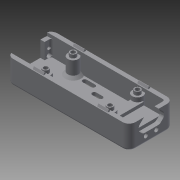
# Autodesk Inventor part: dualBaccable-ucan_fysect
Saved by Autodesk Inventor 2014 SP2 (Build 180246200, 246)
## iProperties
Created: 2025-01-14
Part Number: dualBaccable-ucan_fysect
Material: Generic
Document SubType Name: Sheet Metal
Designer: GauchoHP
Density: 1 g/cm^3
Sheet Metal Rule: Default_mm
Appearance: Default
Author: GauchoHP
Autodesk Inventor part; units mm, degrees
ref_plane "YZ Plane" through (0, 0, 0) normal (1, 0, 0) x (0, 1, 0)
ref_plane "XZ Plane" through (0, 0, 0) normal (0, 1, 0) x (-1, 0, 0)
ref_plane "XY Plane" through (0, 0, 0) normal (0, 0, 1) x (1, 0, 0)
sketch "Sketch1" plane through (0, 0, 0) normal (0, 0, 1) x (1, 0, 0)
  line L0 (-27.1053, 8.3421) -> (24.8947, 8.3421)
  line L1 (27.8947, 5.3421) -> (27.8947, -9.6579)
  line L2 (24.8947, -12.6579) -> (-27.1053, -12.6579)
  line L3 (-30.1053, -9.6579) -> (-30.1053, 5.3421)
  arc A0 (-27.1053, 8.3421) -> (-30.1053, 5.3421) centre (-27.1053, 5.3421) ccw
  arc A1 (27.8947, 5.3421) -> (24.8947, 8.3421) centre (24.8947, 5.3421) ccw
  arc A2 (24.8947, -12.6579) -> (27.8947, -9.6579) centre (24.8947, -9.6579) ccw
  arc A3 (-30.1053, -9.6579) -> (-27.1053, -12.6579) centre (-27.1053, -9.6579) ccw
  point P0 (0, 0)
  point P1 (-30.1053, 8.3421)
  point P2 (27.8947, 8.3421)
  point P3 (-30.1053, -12.6579)
  dimension "d0" = 21
  dimension "d1" = 58
  dimension "d2" = 3
  constraints: 8 end point, 8 point on circle, 8 tangent, 6 point on line, 4 centre point, 3 equal radius, 2 parallel, 1 horizontal, 1 perpendicular
  measures "d0" distance of point (-30.105, -12.658) point (-30.105, 8.342)
  measures "d1" distance of point (-30.105, 8.342) point (27.895, 8.342)
  measures "d2" radius of A0
extrude "Extrusion1" add sketch "Sketch1" along normal blind 2
sketch "Sketch2" plane through (0, 0, 2) normal (0, 0, 1) x (1, 0, 0)
  line L0 (24.8947, 8.3421) -> (-27.1053, 8.3421) projected
  arc A0 (-27.1053, 8.3421) -> (-30.1053, 5.3421) centre (-27.1053, 5.3421) ccw projected
  line L1 (-30.1053, 5.3421) -> (-30.1053, -9.6579) projected
  arc A1 (-30.1053, -9.6579) -> (-27.1053, -12.6579) centre (-27.1053, -9.6579) ccw projected
  line L2 (-27.1053, -12.6579) -> (24.8947, -12.6579) projected
  arc A2 (24.8947, -12.6579) -> (27.8947, -9.6579) centre (24.8947, -9.6579) ccw projected
  line L3 (27.8947, -9.6579) -> (27.8947, 5.3421) projected
  arc A3 (27.8947, 5.3421) -> (24.8947, 8.3421) centre (24.8947, 5.3421) ccw projected
  line L4 (-27.1053, 6.3421) -> (24.8947, 6.3421)
  arc A4 (25.8947, 5.3421) -> (24.8947, 6.3421) centre (24.8947, 5.3421) ccw
  line L5 (25.8947, 5.3421) -> (25.8947, -9.6579)
  arc A5 (24.8947, -10.6579) -> (25.8947, -9.6579) centre (24.8947, -9.6579) ccw
  line L6 (24.8947, -10.6579) -> (-27.1053, -10.6579)
  arc A6 (-28.1053, -9.6579) -> (-27.1053, -10.6579) centre (-27.1053, -9.6579) ccw
  line L7 (-28.1053, -9.6579) -> (-28.1053, 5.3421)
  arc A7 (-27.1053, 6.3421) -> (-28.1053, 5.3421) centre (-27.1053, 5.3421) ccw
  point P0 (0, 0)
  dimension "d5" = 2
  constraints: 8 end point, 8 point on circle, 4 centre point, 7 other
  measures "d5" distance between parallel lines of L4 L0
extrude "Extrusion2" add sketch "Sketch2" along normal blind 9.1
sketch "Sketch4" plane through (-28.1053, -9.6579, 2) normal (1, 0, 0) x (0, 0, -1)
  line L0 (0, 15) -> (0, 0) projected
  line L1 (0, 15) -> (-9.1, 15) projected
  line L2 (0, 0) -> (-9.1, 0) projected
  line L3 (0, 13) -> (-9.5, 13)
  line L4 (-9.5, 13) -> (-9.5, 0)
  line L5 (-9.5, 0) -> (0, 0)
  line L6 (0, 0) -> (0, 13)
  line L7 (-9.5, -1) -> (-7.5, -1)
  line L8 (-7.5, -1) -> (-7.5, 16)
  line L9 (-7.5, 16) -> (-9.5, 16)
  line L10 (-9.5, 16) -> (-9.5, -1)
  point P0 (2, 9.6579)
  dimension "d22" = 9.5
  dimension "d23" = 13
  dimension "d26" = 0
  dimension "d27" = 2
  dimension "d28" = 1
  dimension "d29" = 17
  dimension "d30" = 1
  dimension "d31" = 1
  dimension "d32" = 3
  dimension "d53" = 0
  constraints: 16 end point, 4 parallel, 2 horizontal, 2 perpendicular, 1 point on line
  measures "d22" distance of L5.end L4.end
  measures "d23" distance of L4.end L3.end
  measures "d26" distance between parallel lines of L5 L2
  measures "d27" distance of L8.end L9.end
  measures "d28" distance between parallel lines of L5 L7
  measures "d29" distance of L9.end L7.start
  measures "d30" distance between parallel lines of L9 L1
  measures "d31" distance between parallel lines of L2 L7
  measures "d32" distance between parallel lines of L9 L3
  measures "d53" distance between parallel lines of L4 L10
extrude "Extrusion4" cut sketch "Sketch4" along normal mid plane 10 contours L0 L2 L8 L3 | L8 L3 L10 L9 | L8 L2 L5 L4 L3 | L8 L7 L10 L5 L2
sketch "Sketch5" plane through (0, 0, 2) normal (0, 0, 1) x (1, 0, 0)
  line L0 (-27.1053, -10.6579) -> (24.8947, -10.6579) projected
  line L1 (25.8947, -9.6579) -> (25.8947, 5.3421) projected
  line L2 (24.8947, 6.3421) -> (-27.1053, 6.3421) projected
  line L3 (13.8947, 4.3421) -> (25.8947, 4.3421)
  line L4 (25.8947, 4.3421) -> (25.8947, -8.6579)
  line L5 (25.8947, -8.6579) -> (13.8947, -8.6579)
  line L6 (13.8947, -8.6579) -> (13.8947, 4.3421)
  line L7 (13.8947, -8.6579) -> (16.8947, -8.6579)
  line L8 (16.8947, -8.6579) -> (16.8947, -8.6579)
  line L9 (14.8947, -6.6579) -> (13.8947, -6.6579)
  line L10 (13.8947, -6.6579) -> (13.8947, -8.6579)
  line L11 (13.8947, 4.3421) -> (16.8947, 4.3421)
  line L12 (16.8947, 4.3421) -> (16.8947, 4.3421)
  line L13 (14.8947, 2.3421) -> (13.8947, 2.3421)
  line L14 (13.8947, 2.3421) -> (13.8947, 4.3421)
  arc A0 (14.8947, 2.3421) -> (16.8947, 4.3421) centre (14.8947, 4.3421) ccw
  arc A1 (16.8947, -8.6579) -> (14.8947, -6.6579) centre (14.8947, -8.6579) ccw
  point P0 (0, 0)
  point P1 (16.8947, -6.6579)
  point P2 (16.8947, 2.3421)
  dimension "d35" = 0
  dimension "d36" = 13
  dimension "d37" = 2
  dimension "d38" = 2
  dimension "d39" = 12
  dimension "d152" = 3
  dimension "d153" = 2
  dimension "d154" = 3
  dimension "d155" = 2
  dimension "d156" = 2
  constraints: 24 end point, 6 parallel, 4 point on circle, 4 point on line, 4 tangent, 3 horizontal, 3 perpendicular, 2 centre point, 1 equal radius
  measures "d35" distance between parallel lines of L1 L4
  measures "d36" distance of L5.end L3.start
  measures "d37" distance between parallel lines of L2 L3
  measures "d38" distance between parallel lines of L0 L5
  measures "d39" distance of L3.start L3.end
  measures "d152" distance of L9.end point (16.895, -6.658)
  measures "d153" distance of point (16.895, -6.658) L7.end
  measures "d154" distance of point (16.895, 2.342) L13.end
  measures "d155" distance of L11.end point (16.895, 2.342)
  measures "d156" radius of A0
extrude "Extrusion5" add sketch "Sketch5" along normal blind 4 contours L5 A1 L9 L6 L13 A0 L3 L1
sketch "Sketch6" plane through (0, 0, 2) normal (0, 0, 1) x (1, 0, 0)
  line L0 (25.8947, 4.3421) -> (25.8947, 5.3421) projected
  line L1 (24.8947, 6.3421) -> (-27.1053, 6.3421) projected
  line L2 (-27.1053, -10.6579) -> (24.8947, -10.6579) projected
  line L3 (25.8947, -9.6579) -> (25.8947, -8.6579) projected
  circle A0 centre (14.8947, 4.3421) radius 2.5
  circle A1 centre (14.8947, -8.6579) radius 2.5
  circle A2 centre (14.8947, 4.3421) radius 1
  circle A3 centre (14.8947, -8.6579) radius 1
  circle A4 centre (-15.6053, 4.3421) radius 2.5
  circle A5 centre (-15.6053, -8.6579) radius 2.5
  circle A6 centre (-15.6053, 4.3421) radius 1
  circle A7 centre (-15.6053, -8.6579) radius 1
  point P0 (0, 0)
  dimension "d42" = 5
  dimension "d43" = 5
  dimension "d44" = 11
  dimension "d45" = 11
  dimension "d46" = 2
  dimension "d47" = 2
  dimension "d48" = 13
  dimension "d49" = 2
  dimension "d50" = 2
  dimension "d61" = 5
  dimension "d62" = 5
  dimension "d63" = 2
  dimension "d64" = 2
  dimension "d65" = 13
  dimension "d66" = 2
  dimension "d67" = 30.5
  constraints: 8 centre point, 4 coincident
  measures "d42" diameter of A0
  measures "d43" diameter of A1
  measures "d44" distance from line of A1.centre L3
  measures "d45" distance from line of L0 A0.centre
  measures "d46" diameter of A2
  measures "d47" diameter of A3
  measures "d48" distance of A0.centre A1.centre
  measures "d49" distance from line of L1 A2.centre
  measures "d50" distance from line of L2 A1.centre
  measures "d61" diameter of A4
  measures "d62" diameter of A5
  measures "d63" diameter of A6
  measures "d64" diameter of A7
  measures "d65" distance of A4.centre A5.centre
  measures "d66" distance from line of L1 A6.centre
  measures "d67" distance of A0.centre A4.centre
extrude "Extrusion6" add sketch "Sketch6" along normal blind 7.5
sketch "Sketch7" plane through (14.8947, -8.6579, 2) normal (0, 0, 1) x (1, 0, 0)
  circle A0 centre (0, 0) radius 1 projected
  point P0 (-14.8947, 8.6579)
extrude "Extrusion7" cut sketch "Sketch7" against normal blind 7
sketch "Sketch8" plane through (14.8947, 4.3421, 2) normal (0, 0, 1) x (1, 0, 0)
  circle A0 centre (0, 0) radius 1 projected
  point P0 (-14.8947, -4.3421)
extrude "Extrusion8" cut sketch "Sketch8" against normal blind 7
sketch "Sketch9" plane through (-15.6053, 4.3421, 2) normal (0, 0, 1) x (1, 0, 0)
  circle A0 centre (0, 0) radius 1 projected
  point P0 (15.6053, -4.3421)
extrude "Extrusion9" cut sketch "Sketch9" against normal blind 7
sketch "Sketch10" plane through (-15.6053, -8.6579, 2) normal (0, 0, 1) x (1, 0, 0)
  circle A0 centre (0, 0) radius 1 projected
  point P0 (15.6053, 8.6579)
extrude "Extrusion10" cut sketch "Sketch10" against normal blind 7
sketch "Sketch11" plane through (25.8947, -9.6579, 11.1) normal (-1, 0, 0) x (0, 0, 1)
  line L0 (-9.1, 0) -> (0, 0) projected
  line L1 (-9.1, 15) -> (0, 15) projected
  line L2 (0, 11.0554) -> (-1.9108, 12.9662)
  line L3 (-4.1682, 13.552) -> (-3.3251, 13.552)
  arc A0 (-4.1682, 13.552) -> (-5.1824, 12.9662) centre (-3.7189, 11.6031) ccw
  arc A1 (-6.0108, 12.1378) -> (-6.5966, 10.7236) centre (-4.5966, 10.7236) ccw
  line L4 (-5.1824, 12.9662) -> (-6.0108, 12.1378)
  arc A2 (-6.5966, 4.3804) -> (-6.0108, 2.9662) centre (-4.5966, 4.3804) ccw
  line L5 (-6.0108, 2.9662) -> (-5.1824, 2.1378)
  line L6 (-3.3251, 1.552) -> (-4.1682, 1.552)
  line L7 (-1.9108, 2.1378) -> (0, 4.0486)
  arc A3 (-5.1824, 2.1378) -> (-4.1682, 1.552) centre (-3.7189, 3.5009) ccw
  line L8 (-6.5966, 10.7236) -> (-6.5966, 4.3804)
  line L9 (-5.1, 1) -> (-9.1, 1) projected
  line L10 (-5.1, 14) -> (-5.1, 1) projected
  line L11 (-5.1, 1) -> (-6.6, 1)
  line L12 (0, 15) -> (0, 0) projected
  line L13 (0, 11.0554) -> (0, 4.0486)
  arc A4 (-1.9108, 12.9662) -> (-3.3251, 13.552) centre (-3.3251, 11.552) ccw
  arc A5 (-3.3251, 1.552) -> (-1.9108, 2.1378) centre (-3.3251, 3.552) ccw
  point P0 (-11.1, 9.6579)
  point P1 (-0.4966, 11.552)
  point P2 (-0.4966, 3.552)
  point P3 (-2.4966, 1.552)
  point P4 (-2.4966, 13.552)
  dimension "d72" = 1.448
  dimension "d73" = 1.552
  dimension "d77" = 1.5
  dimension "d78" = 1.4966
  dimension "d148" = 6.5966
  dimension "d149" = 12
  dimension "d150" = 2
  constraints: 18 end point, 12 point on circle, 9 point on line, 6 centre point, 6 tangent, 1 collinear, 1 equal radius
  measures "d72" distance between parallel lines of L1 L3
  measures "d73" distance between parallel lines of L0 L6
  measures "d77" distance of L9.start L11.end
  measures "d78" distance between parallel lines of L10 L8
  measures "d148" distance between parallel lines of L13 L8
  measures "d149" distance between parallel lines of L3 L6
  measures "d150" radius of A4
extrude "Extrusion11" cut sketch "Sketch11" against normal blind 7
sketch "Sketch12" plane through (27.8947, -9.6579, 0) normal (1, 0, 0) x (0, 0, -1)
  line L0 (0, 15) -> (0, 0) projected
  line L1 (0, 15) -> (-11.1, 15) projected
  line L2 (0, 0) -> (-11.1, 0) projected
  circle A0 centre (-3, 10) radius 1
  circle A1 centre (-3, 5) radius 1
  point P0 (0, 9.6579)
  dimension "d79" = 2
  dimension "d80" = 2
  dimension "d81" = 3
  dimension "d82" = 3
  dimension "d83" = 5
  dimension "d84" = 5
  constraints: 2 centre point
  measures "d79" diameter of A0
  measures "d80" diameter of A1
  measures "d81" distance from line of L0 A1.centre
  measures "d82" distance from line of L0 A0.centre
  measures "d83" distance from line of L2 A1.centre
  measures "d84" distance from line of L1 A0.centre
extrude "Extrusion12" cut sketch "Sketch12" against normal blind 15
sketch "Sketch13" plane through (0, 0, 2) normal (0, 0, 1) x (1, 0, 0)
  line L0 (25.8947, 4.3421) -> (25.8947, 5.3421) projected
  line L1 (13.3947, 6.3421) -> (-14.1053, 6.3421) projected
  line L2 (-2.6053, 2.3421) -> (0.3947, 2.3421)
  line L3 (1.3947, 1.3421) -> (1.3947, 1.3421)
  line L4 (0.3947, 0.3421) -> (-2.6053, 0.3421)
  line L5 (-3.6053, 1.3421) -> (-3.6053, 1.3421)
  arc A0 (-2.6053, 2.3421) -> (-3.6053, 1.3421) centre (-2.6053, 1.3421) ccw
  arc A1 (1.3947, 1.3421) -> (0.3947, 2.3421) centre (0.3947, 1.3421) ccw
  arc A2 (0.3947, 0.3421) -> (1.3947, 1.3421) centre (0.3947, 1.3421) ccw
  arc A3 (-3.6053, 1.3421) -> (-2.6053, 0.3421) centre (-2.6053, 1.3421) ccw
  line L6 (-10.1053, 5.3421) -> (-6.1053, 5.3421)
  line L7 (-5.1053, 4.3421) -> (-5.1053, 4.3421)
  line L8 (-6.1053, 3.3421) -> (-10.1053, 3.3421)
  line L9 (-11.1053, 4.3421) -> (-11.1053, 4.3421)
  arc A4 (-10.1053, 5.3421) -> (-11.1053, 4.3421) centre (-10.1053, 4.3421) ccw
  arc A5 (-5.1053, 4.3421) -> (-6.1053, 5.3421) centre (-6.1053, 4.3421) ccw
  arc A6 (-6.1053, 3.3421) -> (-5.1053, 4.3421) centre (-6.1053, 4.3421) ccw
  arc A7 (-11.1053, 4.3421) -> (-10.1053, 3.3421) centre (-10.1053, 4.3421) ccw
  point P0 (0, 0)
  point P1 (-3.6053, 2.3421)
  point P2 (1.3947, 2.3421)
  point P3 (-3.6053, 0.3421)
  point P4 (1, 1)
  point P5 (-11.1053, 5.3421)
  point P6 (-5.1053, 5.3421)
  point P7 (-11.1053, 3.3421)
  dimension "d87" = 24.5
  dimension "d88" = 5
  dimension "d89" = 4
  dimension "d90" = 2
  dimension "d91" = 1
  dimension "d97" = 6
  dimension "d98" = 2
  dimension "d99" = 1
  dimension "d100" = 1
  dimension "d101" = 32
  constraints: 16 end point, 16 point on circle, 16 tangent, 12 point on line, 8 centre point, 6 equal radius, 4 parallel, 2 horizontal, 2 perpendicular
  measures "d87" distance between parallel lines of L3 L0
  measures "d88" distance of point (-3.605, 2.342) point (1.395, 2.342)
  measures "d89" distance between parallel lines of L1 L2
  measures "d90" distance of point (-3.605, 0.342) point (-3.605, 2.342)
  measures "d91" radius of A0
  measures "d97" distance of point (-11.105, 5.342) point (-5.105, 5.342)
  measures "d98" distance of point (-11.105, 3.342) point (-11.105, 5.342)
  measures "d99" radius of A4
  measures "d100" distance between parallel lines of L1 L6
  measures "d101" distance from line of L0 A5.centre
extrude "Extrusion13" cut sketch "Sketch13" against normal blind 10
chamfer "Chamfer2" distance 0.5 angle 45 8 edges at (-1.1053, 0.3421, 0) (1.3947, 1.3421, 0) (-1.1053, 2.3421, 0) (-3.6053, 1.3421, 0) (-8.1053, 3.3421, 0) (-5.1053, 4.3421, 0) (-8.1053, 5.3421, 0) (-11.1053, 4.3421, 0)
sketch "Sketch15" plane through (0, 0, 11.1) normal (0, 0, 1) x (1, 0, 0)
  line L0 (24.8947, 8.3421) -> (-27.1053, 8.3421) projected
  line L1 (-13.1053, 7.4421) -> (-18.1053, 7.4421)
  line L2 (-18.1053, 7.4421) -> (-18.1053, 7.2421)
  line L3 (-18.1053, 7.2421) -> (-13.1053, 7.2421)
  line L4 (-13.1053, 7.2421) -> (-13.1053, 7.4421)
  circle A0 centre (-15.6053, 4.3421) radius 1 projected
  line L5 (12.3947, 7.4421) -> (17.3947, 7.4421)
  line L6 (17.3947, 7.4421) -> (17.3947, 7.2421)
  line L7 (17.3947, 7.2421) -> (12.3947, 7.2421)
  line L8 (12.3947, 7.2421) -> (12.3947, 7.4421)
  circle A1 centre (14.8947, 4.3421) radius 1 projected
  line L9 (12.3947, -11.5579) -> (17.3947, -11.5579)
  line L10 (17.3947, -11.5579) -> (17.3947, -11.7579)
  line L11 (17.3947, -11.7579) -> (12.3947, -11.7579)
  line L12 (12.3947, -11.7579) -> (12.3947, -11.5579)
  circle A2 centre (14.8947, -8.6579) radius 1 projected
  line L13 (24.8947, -12.6579) -> (-27.1053, -12.6579) projected
  line L14 (-18.1053, -11.5579) -> (-13.1053, -11.5579)
  line L15 (-13.1053, -11.5579) -> (-13.1053, -11.7579)
  line L16 (-13.1053, -11.7579) -> (-18.1053, -11.7579)
  line L17 (-18.1053, -11.7579) -> (-18.1053, -11.5579)
  circle A3 centre (-15.6053, -8.6579) radius 1 projected
  line L18 (-32.7112, 10.999) -> (37.2662, 10.999)
  line L19 (37.2662, 10.999) -> (37.2662, -17.3702)
  line L20 (37.2662, -17.3702) -> (-32.7112, -17.3702)
  line L21 (-32.7112, -17.3702) -> (-32.7112, 10.999)
  point P0 (0, 0)
  dimension "d104" = 0.2
  dimension "d105" = 0.9
  dimension "d107" = 5
  dimension "d108" = 2.5
  dimension "d109" = 5
  dimension "d110" = 0.2
  dimension "d111" = 0.9
  dimension "d112" = 2.5
  dimension "d113" = 5
  dimension "d114" = 0.2
  dimension "d115" = 2.5
  dimension "d116" = 0.9
  dimension "d117" = 5
  dimension "d118" = 0.2
  dimension "d119" = 0.9
  dimension "d120" = 2.5
  constraints: 40 end point, 10 parallel, 5 horizontal, 5 perpendicular
  measures "d104" distance of L1.end L2.end
  measures "d105" distance between parallel lines of L0 L1
  measures "d107" distance of L1.start L1.end
  measures "d108" distance from line of L4 A0.centre
  measures "d109" distance of L6.end L7.end
  measures "d110" distance of L5.end L6.end
  measures "d111" distance between parallel lines of L0 L5
  measures "d112" distance from line of A1.centre L6
  measures "d113" distance of L10.end L11.end
  measures "d114" distance of L9.end L10.end
  measures "d115" distance from line of A2.centre L12
  measures "d116" distance between parallel lines of L13 L11
  measures "d117" distance of L15.end L16.end
  measures "d118" distance of L14.end L15.end
  measures "d119" distance between parallel lines of L16 L13
  measures "d120" distance from line of A3.centre L17
extrude "Extrusion14" add sketch "Sketch15" along normal blind 1 contours L4 L3 L2 L1 | L5 L6 L7 L8 | L9 L10 L11 L12 | L14 L15 L16 L17
chamfer "Chamfer3" distance 0.5 distance2 1 1 edges at (-15.6053, -11.7579, 11.1)
chamfer "Chamfer4" distance 0.5 distance2 1 1 edges at (-15.6053, -11.5579, 11.1)
chamfer "Chamfer5" distance 0.5 distance2 1 1 edges at (14.8947, -11.7579, 11.1)
chamfer "Chamfer6" distance 0.5 distance2 1 1 edges at (14.8947, -11.5579, 11.1)
chamfer "Chamfer7" distance 0.5 distance2 1 1 edges at (14.8947, 7.4421, 11.1)
chamfer "Chamfer8" distance 0.5 distance2 1 1 edges at (14.8947, 7.2421, 11.1)
chamfer "Chamfer9" distance 0.5 distance2 1 1 edges at (-15.6053, 7.4421, 11.1)
chamfer "Chamfer10" distance 0.5 distance2 1 1 edges at (-15.6053, 7.2421, 11.1)
fillet "Fillet2" radius 1 8 edges at (-29.2266, 7.4634, 0) (-1.1053, 8.3421, 0) (27.0161, 7.4634, 0) (27.8947, -2.1579, 0) (27.0161, -11.7792, 0) (-1.1053, -12.6579, 0) (-29.2266, -11.7792, 0) (-30.1053, -2.1579, 0)
sketch "Sketch16" plane through (0, 0, 6) normal (0, 0, 1) x (1, 0, 0)
  arc A0 (13.8947, 2.0508) -> (17.3947, 4.3421) centre (14.8947, 4.3421) ccw projected
  line L0 (13.8947, 2.0508) -> (13.8947, -6.3666) projected
  arc A1 (17.3947, -8.6579) -> (13.8947, -6.3666) centre (14.8947, -8.6579) ccw projected
  line L1 (17.3947, -8.6579) -> (25.8947, -8.6579) projected
  line L2 (25.8947, 4.3421) -> (17.3947, 4.3421) projected
  line L3 (17.8947, 4.3421) -> (17.3947, 4.3421)
  line L4 (17.8947, 4.3421) -> (17.8947, -8.6579)
  point P0 (0, 0)
  constraints: 4 end point, 2 point on line, 1 perpendicular
extrude "Extrusion15" add sketch "Sketch16" along normal blind 1.5
sketch "Sketch17" plane through (-28.1053, 3.3421, 2) normal (1, 0, 0) x (0, 0, -1)
  line L0 (0, 2) -> (0, 0) projected
  line L1 (0, 2) -> (-7.5, 2) projected
  circle A0 centre (-1, 2) radius 1
  circle A1 centre (-4, 2) radius 0.75
  point P0 (2, -3.3421)
  dimension "d160" = 0
  dimension "d161" = 1
  dimension "d164" = 1.5
  dimension "d165" = 3
  constraints: 2 centre point, 1 point on line
  measures "d160" distance from line of L1 A0.centre
  measures "d161" distance from line of L0 A0.centre
  measures "d164" diameter of A1
  measures "d165" distance of A0.centre A1.centre
extrude "Extrusion16" cut sketch "Sketch17" along normal mid plane 5
sketch "Sketch18" plane through (0, 0, 9.5) normal (0, 0, 1) x (1, 0, 0)
  circle A0 centre (14.8947, -8.6579) radius 1 projected
  circle A1 centre (14.8947, -8.6579) radius 1.45
  point P0 (0, 0)
  dimension "d166" = 2.9
  constraints: 1 centre point, 1 coincident
  measures "d166" diameter of A1
extrude "Extrusion17" add sketch "Sketch18" along normal blind 1.6
sketch "Sketch19" plane through (0, 0, 9.5) normal (0, 0, 1) x (1, 0, 0)
  circle A0 centre (14.8947, 4.3421) radius 1 projected
  circle A1 centre (14.8947, 4.3421) radius 1.45
  point P0 (0, 0)
  dimension "d169" = 2.9
  constraints: 1 centre point, 1 coincident
  measures "d169" diameter of A1
extrude "Extrusion18" add sketch "Sketch19" along normal blind 1.6
sketch "Sketch20" plane through (0, 0, 9.5) normal (0, 0, 1) x (1, 0, 0)
  circle A0 centre (-15.6053, 4.3421) radius 1 projected
  circle A1 centre (-15.6053, 4.3421) radius 1.45
  point P0 (0, 0)
  dimension "d172" = 2.9
  constraints: 1 centre point, 1 coincident
  measures "d172" diameter of A1
extrude "Extrusion19" add sketch "Sketch20" along normal blind 1.6
sketch "Sketch21" plane through (0, 0, 9.5) normal (0, 0, 1) x (1, 0, 0)
  circle A0 centre (-15.6053, -8.6579) radius 1 projected
  circle A1 centre (-15.6053, -8.6579) radius 1.45
  point P0 (0, 0)
  dimension "d175" = 2.9
  constraints: 1 centre point, 1 coincident
  measures "d175" diameter of A1
extrude "Extrusion20" add sketch "Sketch21" along normal blind 1.6
chamfer "Chamfer11" distance 1.2 angle 45 1 edges at (12.4115, -8.3686, 2)
chamfer "Chamfer12" distance 1.2 angle 45 5 edges at (-15.6053, -6.1579, 2) (-15.6053, 1.8421, 2) (12.4115, 4.0528, 2) (17.1308, 5.4601, 2) (17.1308, -9.7759, 2)
sketch "Sketch22" plane through (0, 0, 0) normal (0, 0, -1) x (-1, 0, 0)
  circle A0 centre (-14.8947, -8.6579) radius 1 projected
  circle A1 centre (-14.8947, 4.3421) radius 1 projected
  circle A2 centre (15.6053, 4.3421) radius 1 projected
  circle A3 centre (15.6053, -8.6579) radius 1 projected
  circle A4 centre (-14.8947, 4.3421) radius 2.5
  circle A5 centre (15.6053, 4.3421) radius 2.5
  circle A6 centre (-14.8947, -8.6579) radius 2.5
  circle A7 centre (15.6053, -8.6579) radius 2.5
  point P0 (0, 0)
  dimension "d178" = 5
  dimension "d179" = 5
  dimension "d180" = 5
  dimension "d181" = 5
  constraints: 4 centre point, 4 coincident
  measures "d178" diameter of A4
  measures "d179" diameter of A5
  measures "d180" diameter of A6
  measures "d181" diameter of A7
extrude "Extrusion21" cut sketch "Sketch22" against normal blind 2.5
equation "\"BendRadius\" = Thickness"
equation "\"BendReliefWidth\" = Thickness"
equation "\"BendReliefDepth\" = 0.5 * Thickness"
equation "\"CornerReliefSize\" = 4 * Thickness"
equation "\"MinimumRemnant\" = 2 * Thickness"
equation "\"TransitionRadius\" = BendRadius"
equation "\"JacobiRadiusSize\" = BendRadius"
equation "\"GapSize\" = Thickness"
equation "\"Thickness\" = 0.5"
body "Solid1"
